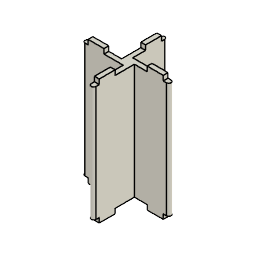
InnerSupport_v5 (Autodesk Fusion 360 design; units mm, degrees)
Autodesk Fusion 360 part; units mm, degrees
sketch "Sketch1" plane through (0, 0, 0) normal (0, 0, 1) x (1, 0, 0)
  line L0 (0, 0) -> (25, 0)
  line L1 (25, 0) -> (25, 3)
  line L2 (25, 3) -> (0, 3)
  line L3 (0, 3) -> (0, 0)
  line L4 (0, 25) -> (-3, 25)
  line L5 (-3, 25) -> (-3, 0)
  line L6 (0, 0) -> (0, 25)
  line L7 (-25, 0) -> (-25, -3)
  line L8 (-25, -3) -> (0, -3)
  line L9 (0, 0) -> (-25, 0)
  line L10 (0, -25) -> (3, -25)
  line L11 (3, -25) -> (3, 0)
  line L12 (0, 0) -> (0, -25)
  dimension "d1" = 25
  dimension "d2" = 3
  dimension "d5" = 0
  dimension "d6" = 0
  dimension "d8" = 360
  constraint horizontal L0
  constraint vertical L1
  constraint horizontal L2
  constraint vertical L3
  constraint coincident L0.start L3.end
  measures "d1" distance of L0.start L0.end
  measures "d2" distance of L0.start L2.end
extrude "Extrude1" add sketch "Sketch1" along normal blind 72
move_face "OffsetFaces1" offset -0.5 4 faces at (10.3333, 0, 48) (0, 10.3333, 48) (0, -10.3333, 48) (-10.3333, 0, 48)
move_face "OffsetFaces2" offset 0.5 4 faces at (-3, 16.5, 24) (-16.5, -3, 24) (3, -16.5, 24) (16.5, 3, 24)
fillet "Fillet1" radius 1.5 8 edges at (3.5, -25, 36) (0.5, -25, 36) (25, 0.5, 36) (25, 3.5, 36) (-25, -3.5, 36) (-25, -0.5, 36) (-3.5, 25, 36) (-0.5, 25, 36)
sketch "Sketch2" plane through (0, 0, 72) normal (0, 0, 1) x (-1, 0, 0)
  arc A0 (0.5, -23.5) -> (3.5, -23.5) centre (2, -23.5) ccw
  line L0 (3.5, -23.5) -> (3.5, 0.5)
  line L1 (3.5, 0.5) -> (23.5, 0.5)
  arc A1 (23.5, 0.5) -> (23.5, 3.5) centre (23.5, 2) ccw
  line L2 (23.5, 3.5) -> (-0.5, 3.5)
  line L3 (-0.5, 3.5) -> (-0.5, 23.5)
  arc A2 (-0.5, 23.5) -> (-3.5, 23.5) centre (-2, 23.5) ccw
  line L4 (-3.5, 23.5) -> (-3.5, -0.5)
  line L5 (-3.5, -0.5) -> (-23.5, -0.5)
  arc A3 (-23.5, -0.5) -> (-23.5, -3.5) centre (-23.5, -2) ccw
  line L6 (-23.5, -3.5) -> (0.5, -3.5)
  line L7 (0.5, -3.5) -> (0.5, -23.5)
  line L8 (-3.5, 21.5) -> (-0.5, 21.5)
  line L9 (-3.5, 11.5) -> (-0.5, 11.5)
  line L10 (-21.5, -3.5) -> (-21.5, -0.5)
  line L11 (-11.5, -3.5) -> (-11.5, -0.5)
  line L12 (3.5, -21.5) -> (0.5, -21.5)
  line L13 (3.5, -11.5) -> (0.5, -11.5)
  line L14 (21.5, 3.5) -> (21.5, 0.5)
  line L15 (11.5, 3.5) -> (11.5, 0.5)
  dimension "d22" = 10
  dimension "d23" = 8
  dimension "d25" = 360
  constraint coincident L4 L8.start
  constraint coincident L3 L8.end
  constraint perpendicular L3 L8
  constraint coincident L4 L9.start
  constraint coincident L3 L9.end
  constraint perpendicular L3 L9
  measures "d22" distance of L8 L9
  measures "d23" distance of L2 L9
extrude "Extrude2" add sketch "Sketch2" along normal blind 3 contours L0 L7 L12 L13 | L5 L6 L10 L11 | L1 L2 L14 L15 | L3 L4 L8 L9
extrude "Extrude3" add sketch "Sketch2" against normal blind 75 contours L0 L7 L12 L13 | L5 L6 L10 L11 | L1 L2 L14 L15 | L3 L4 L8 L9
